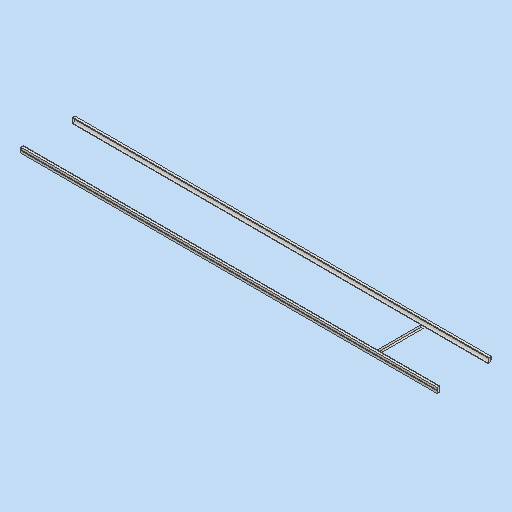
# Autodesk Inventor part: esteira
Saved by Autodesk Inventor 2025.3 (Build 293356000, 356)
## iProperties
Created: 2025-10-23
Part Number: esteira
Material: Genérico
Document SubType Name: Modeling
Designer: gabriel.bispo
Density: 1 g/cm^3
Appearance: Padrão
Author: gabriel.bispo
Autodesk Inventor part; units mm, degrees
ref_plane "YZ Plane" through (0, 0, 0) normal (1, 0, 0) x (0, 1, 0)
ref_plane "XZ Plane" through (0, 0, 0) normal (0, 1, 0) x (-1, 0, 0)
ref_plane "XY Plane" through (0, 0, 0) normal (0, 0, 1) x (1, 0, 0)
sketch "Esboço1" plane through (0, 0, 0) normal (0, 1, 0) x (-1, 0, 0)
  line L0 (0, 0) -> (9550, 0)
  line L1 (0, 0) -> (0, -60)
  line L2 (0, -60) -> (9550, -60)
  line L3 (9550, 0) -> (9550, -60)
  line L4 (0, 0) -> (0, -1180)
  line L5 (0, -1180) -> (9550, -1180)
  line L6 (0, -1180) -> (0, -1240)
  line L7 (0, -1180) -> (60, -1180) construction
  line L8 (0, -1240) -> (9550, -1240)
  line L9 (9550, -1180) -> (9550, -1240)
  line L10 (0, -60) -> (154, -60)
  line L11 (154.5, -60.0033) -> (154.5, -118.0033)
  line L12 (0, -1180) -> (1550, -1180)
  line L13 (0, -60) -> (1550, -60)
  line L14 (1550, -60) -> (1550, -60)
  line L15 (1621.1615, -1180) -> (1614.2387, -1180)
  line L16 (1550, -1180) -> (1550, -60)
  line L17 (1550, -60) -> (1549.5, -60)
  line L18 (1550, -1180) -> (1550, -1180.5)
  line L19 (1550, -1180) -> (1549.5, -1180)
  line L20 (1549.5, -1180) -> (1549.5, -60)
  dimension "d0" = 9550
  dimension "d1" = 60
  dimension "d3" = 1180
  dimension "d5" = 60
  dimension "d7" = 9550
  dimension "d8" = 154
  dimension "d15" = 1550
  dimension "d16" = 1550
  dimension "d19" = 0.5
  dimension "d21" = 0.5
  constraints: 42 end point, 8 point on line, 5 perpendicular, 4 horizontal, 2 vertical, 1 collinear
  measures "d0" distance of L0.start L0.end
  measures "d1" distance of L0.start L1.end
  measures "d3" distance of L0.start L4.end
  measures "d5" distance of L4.end L6.end
  measures "d7" distance of L6.end L8.end
  measures "d8" distance of L1.end L10.end
  measures "d15" distance of L4.end L12.end
  measures "d16" distance of L1.end L13.end
  measures "d19" distance of L14.end L17.end
  measures "d21" distance of L12.end L19.end
extrude "Extrusão1" add sketch "Esboço1" along normal blind 120 contours L0 L3 L2 L1 | L5 L9 L8 L6
sketch "Esboço4" plane through (-9550, 0, -1180) normal (0, 0, 1) x (1, 0, 0)
  line L0 (9549.5, 119.5) -> (9549.5, 0.5)
  line L1 (0.5, 119.5) -> (0.5, 0.5)
  line L2 (0.5, 0.5) -> (9549.5, 0.5)
  line L3 (9549.5, 119.5) -> (0.5, 119.5)
  point P0 (9550, 0)
  constraints: 8 end point, 2 perpendicular
extrude "Extrusão2" add sketch "Esboço1" against normal blind 50 contours L16 L5 L20 L2
extrude "Extrusão3" cut sketch "Esboço4" against normal blind 59.5
fillet "Arredondamento1" radius 50 1 edges at (-4775, 119.5, -1239.5)
fillet "Arredondamento2" radius 50 2 edges at (-4775, 0.5, -1239.5) (-4775, 0, -1240)
sketch "Esboço5" plane through (0, 120, -60) normal (0, 0, -1) x (-1, 0, 0)
  line L0 (0, -120) -> (0.5, -120)
  line L1 (0.5, -0.5) -> (0.5, -116.4149)
  line L2 (9549.4996, -119.5) -> (9549.4996, -0.5)
  line L3 (9549.4996, -119.5) -> (0.5, -116.4149)
  line L4 (0.5, -0.5) -> (9549.4996, -0.5)
  dimension "d39" = 0.5
  constraints: 10 end point, 1 horizontal, 1 perpendicular, 1 vertical
  measures "d39" distance of L0.start L0.end
extrude "Extrusão4" cut sketch "Esboço5" against normal blind 59.5
fillet "Arredondamento3" radius 50 1 edges at (-4774.9998, 119.5, -0.5)
fillet "Arredondamento4" radius 50 1 edges at (-4774.9998, 2.0425, -0.5)
sketch "Esboço6" plane through (-1549.5, 0, -60) normal (1, 0, 0) x (0, 0, -1)
  line L0 (0, -50) -> (1120.0002, -50)
  line L1 (0, -50) -> (0, -49.5)
  line L2 (0, -49.5) -> (1120.0002, -49.5)
  line L3 (1120.0002, -49.5) -> (1120.0002, -50)
  point P0 (-60, 0)
  dimension "d52" = 0.5
  dimension "d53" = 90
  constraints: 8 end point, 1 perpendicular, 1 vertical
  measures "d52" distance of L0.start L1.end
  measures "d53" angle of L1 L2
extrude "Extrusão5" add sketch "Esboço6" along normal blind 50
